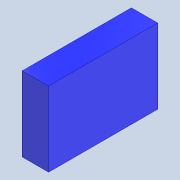
# Autodesk Inventor part: Mangas_soporte_molde
Saved by Autodesk Inventor 2021 (Build 250183000, 183)
## iProperties
Created: 2021-04-17
Part Number: Mangas_soporte_molde
Material: Genérico
Document SubType Name: Modeling
Designer: Admin
Density: 1 g/cm^3
Appearance: Azul - Pintura mural - Brillante
Author: Admin
Autodesk Inventor part; units mm, degrees
ref_plane "YZ Plane" through (0, 0, 0) normal (1, 0, 0) x (0, 1, 0)
ref_plane "XZ Plane" through (0, 0, 0) normal (0, 1, 0) x (-1, 0, 0)
ref_plane "XY Plane" through (0, 0, 0) normal (0, 0, 1) x (1, 0, 0)
sketch "Boceto1" plane through (0, 0, 0) normal (0, 0, 1) x (1, 0, 0)
  line L0 (0, 0) -> (6.4, 0)
  line L1 (6.4, 0) -> (6.4, 25.4)
  line L2 (6.4, 25.4) -> (0, 25.4)
  line L3 (0, 25.4) -> (0, 0)
  line L4 (-2, 0) -> (-2, 27.4)
  line L5 (-2, 27.4) -> (8.4, 27.4)
  line L6 (8.4, 27.4) -> (8.4, -2)
  line L7 (8.4, -2) -> (-2, -2)
  line L8 (-2, -2) -> (-2, 0)
  dimension "d0" = 6.4
  dimension "d1" = 25.4
  dimension "d2" = 2
  dimension "d3" = 27.4
  dimension "d4" = 10.4
  dimension "d5" = 29.4
  constraints: 18 end point, 5 perpendicular, 2 parallel, 1 horizontal, 1 point on line, 1 vertical
  measures "d0" distance of L2.end L1.end
  measures "d1" distance of L1.end L0.end
  measures "d2" distance of L0.start L4.start
  measures "d3" distance of L4.start L4.end
  measures "d4" distance of L4.end L5.end
  measures "d5" distance of L5.end L6.end
extrude "Extrusión1" add sketch "Boceto1" along normal blind 41
sketch "Boceto2" plane through (0, 0, 41) normal (0, 0, 1) x (1, 0, 0)
  line L0 (-2, -2) -> (8.4, -2) projected
  line L1 (-2, -2) -> (8.4, -2)
  line L2 (8.4, -2) -> (8.4, 27.4)
  line L3 (8.4, 27.4) -> (-2, 27.4)
  line L4 (-2, 27.4) -> (-2, -2)
  point P0 (0, 0)
  constraints: 8 end point, 2 parallel, 1 horizontal, 1 perpendicular
extrude "Extrusión2" add sketch "Boceto2" along normal blind 2
